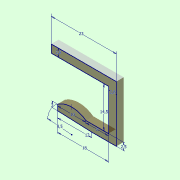
# Autodesk Inventor part: Cuvette_retainer
Saved by Autodesk Inventor 2015 (Build 190159000, 159)
## iProperties
Created: 2015-05-25
Part Number: Cuvette_retainer
Material: Generic
Document SubType Name: Modeling
Designer: Openlab
Density: 1 g/cm^3
Appearance: Polycarbonate - Smoked
Author: Openlab
Autodesk Inventor part; units mm, degrees
ref_plane "YZ Plane" through (0, 0, 0) normal (1, 0, 0) x (0, 1, 0)
ref_plane "XZ Plane" through (0, 0, 0) normal (0, 1, 0) x (-1, 0, 0)
ref_plane "XY Plane" through (0, 0, 0) normal (0, 0, 1) x (1, 0, 0)
sketch "Sketch1" plane through (0, 0, 0) normal (0, 1, 0) x (-1, 0, 0)
  line L0 (0, 0) -> (23, 0)
  line L1 (23, 0) -> (23, -2.8)
  line L2 (0, 0) -> (0, -19.8)
  line L3 (0, -19.8) -> (8.8, -19.8)
  line L4 (20.8, -19.3) -> (20.8, -17.3)
  line L5 (10.8, -17.3) -> (2.8, -17.3)
  line L6 (2.8, -17.3) -> (2.8, -2.8)
  line L7 (2.8, -2.8) -> (23, -2.8)
  arc A0 (20.8, -17.3) -> (10.8, -17.3) centre (15.8, -24.1739) ccw
  line L8 (8.8, -19.8) -> (20.8, -19.3)
  point P0 (15.8, -15.6739)
  dimension "d1" = 2.8
  dimension "d3" = 2.8
  dimension "d4" = 23
  dimension "d9" = 12
  dimension "d10" = 2
  dimension "d11" = 10
  dimension "d12" = 8
  dimension "d13" = 14.5
  dimension "d14" = 8.5
  dimension "d15" = 18
  dimension "d16" = 2.5
  constraints: 18 end point, 4 perpendicular, 3 point on circle, 2 vertical, 1 centre point, 1 horizontal
  measures "d1" distance of L0.end L1.end
  measures "d3" distance between parallel lines of L2 L6
  measures "d4" distance of L0.start L0.end
  measures "d9" horizontal distance of L4.start L3.end
  measures "d10" distance of L4.start L4.end
  measures "d11" distance of L5.start L4.end
  measures "d12" distance of L5.start L5.end
  measures "d13" distance of L5.end L6.end
  measures "d14" radius of A0
  measures "d15" distance between parallel lines of L6 L4
  measures "d16" distance between parallel lines of L5 L3
extrude "Extrusion1" add sketch "Sketch1" along normal blind 2.6
body "Solid1"
